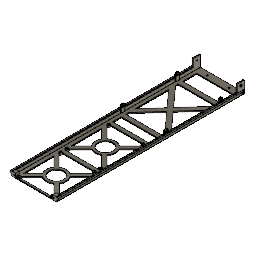
1-CBA_slide_tray_assembly_v11 (Autodesk Fusion 360 design; units mm, degrees)
Autodesk Fusion 360 part; units mm, degrees
sketch "Main Profile" plane through (0, 0, 0) normal (0, 1, 0) x (1, 0, 0)
  line L0 (0, 0) -> (62.1, 0)
  line L1 (62.1, 0) -> (62.1, -5.4)
  line L2 (62.1, -5.4) -> (66.55, -5.4)
  line L3 (66.55, -5.4) -> (66.55, -11.15)
  line L4 (66.55, -11.15) -> (62.1, -11.15)
  line L5 (62.1, -11.15) -> (62.1, -11.6)
  line L6 (62.1, -11.6) -> (58.7, -11.6)
  line L7 (58.7, -11.6) -> (58.7, -2.95)
  line L8 (58.7, -2.95) -> (0, -2.95)
  line L9 (0, -2.95) -> (0, 0) construction
  line L10 (0, 0) -> (-62.1, 0)
  line L11 (-62.1, 0) -> (-62.1, -5.4)
  line L12 (-62.1, -5.4) -> (-66.55, -5.4)
  line L13 (-66.55, -5.4) -> (-66.55, -11.15)
  line L14 (-66.55, -11.15) -> (-62.1, -11.15)
  line L15 (-62.1, -11.15) -> (-62.1, -11.6)
  line L16 (-62.1, -11.6) -> (-58.7, -11.6)
  line L17 (-58.7, -11.6) -> (-58.7, -2.95)
  line L18 (-58.7, -2.95) -> (0, -2.95)
  line L19 (60.6, -12.45) -> (50.6, -12.45)
  line L20 (50.6, -12.45) -> (50.6, -2.95)
  line L21 (60.6, -11.6) -> (60.6, -12.45)
  circle A0 centre (54.4, -6.11) radius 1.75
  circle A1 centre (54.4, -6.11) radius 2.5
  circle A2 centre (-54.4, -6.11) radius 1.75
  circle A3 centre (-54.4, -6.11) radius 2.5
  line L22 (-50.6, -12.45) -> (-50.6, -2.95)
  line L23 (-60.6, -12.45) -> (-50.6, -12.45)
  line L24 (-60.6, -11.6) -> (-60.6, -12.45)
  dimension "d1" = 2.95
  dimension "d2" = 5.75
  dimension "d3" = 5.4
  dimension "d4" = 4.45
  dimension "d5" = 62.1
  dimension "d6" = 11.6
  dimension "d7" = 3.4
  dimension "d10" = 10
  dimension "d11" = 9.5
  dimension "d12" = 50.6
  dimension "d13" = 3.5
  dimension "d14" = 5
  dimension "d15" = 3.16
  dimension "d16" = 54.4
  constraint coincident L0.start L9.end
  constraint horizontal L0
  constraint perpendicular L0 L1
  constraint perpendicular L1 L2
  constraint perpendicular L2 L3
  constraint perpendicular L3 L4
  constraint perpendicular L4 L5
  constraint perpendicular L5 L6
  constraint perpendicular L6 L7
  constraint perpendicular L7 L8
  constraint vertical L9
  constraint symmetric L0.start L9 L10.start
  constraint symmetric L0.end L9 L10.end
  constraint symmetric L1.end L9 L11.end
  constraint symmetric L2.end L9 L12.end
  constraint symmetric L3.end L9 L13.end
  constraint symmetric L4.end L9 L14.end
  constraint symmetric L5.end L9 L15.end
  constraint symmetric L6.end L9 L16.end
  constraint symmetric L7.end L9 L17.end
  constraint symmetric L8.end L9 L18.end
  constraint horizontal L19
  constraint vertical L20
  constraint vertical L21
  constraint coincident L6 L21.start
  constraint coincident L8 L20.end
  constraint concentric A0 A1
  constraint collinear L1 L5
  constraint symmetric L9 L19.start L23.start
  constraint symmetric L9 L19.end L22.start
  constraint symmetric L9 L20.end L22.end
  constraint symmetric L9 L21.start L24.start
  constraint symmetric L9 A0 A2
  constraint symmetric L9 A1 A3
  measures "d1" distance of L0 L8
  measures "d2" distance of L2 L4
  measures "d3" distance of L0 L2
  measures "d4" distance of L1 L3
  measures "d5" distance of L0.start L1
  measures "d6" distance of L0 L6
  measures "d7" distance of L1 L7
  measures "d10" distance of L19.start L19.end
  measures "d11" distance of L8 L19
  measures "d12" distance of L0.start L20
  measures "d13" diameter of A0
  measures "d14" diameter of A1
  measures "d15" distance of L8 A0.centre
  measures "d16" horizontal distance of L8.end A0.centre
extrude "Extrude1" add sketch "Main Profile" along normal blind 515.25 contours L0 L1 L2 L3 L4 L5 L6 L7 L8 L10 L11 L12 L13 L14 L15 L16 L17 L18
extrude "Extrude2" add sketch "Main Profile" along normal blind 10 contours L6 L7 L8 L19 L20 L21 | L16 L17 L18 L22 L23 L24
extrude "Extrude3" add sketch "Main Profile" along normal blind 5 contours A1 | A3
sketch "Solver says NO" plane through (0, 0, 0) normal (0, 0, 1) x (1, 0, 0)
  circle A0 centre (45.9, 4.2) radius 4
  circle A1 centre (45.9, 4.2) radius 2.5
  circle A2 centre (45.9, 4.2) radius 1.75
  circle A3 centre (0, 61) radius 20
  circle A4 centre (0, 61) radius 27.5
  circle A5 centre (-46.134, 4.2) radius 1.75
  circle A6 centre (-46.134, 4.2) radius 2.5
  circle A7 centre (-46.134, 4.2) radius 4
  circle A8 centre (45.9, 119.158) radius 1.75
  circle A9 centre (45.9, 119.158) radius 2.5
  circle A10 centre (45.9, 119.158) radius 4
  circle A11 centre (-46.134, 119.158) radius 1.75
  circle A12 centre (-46.134, 119.158) radius 2.5
  circle A13 centre (-46.134, 119.158) radius 4
  line L0 (-42.261, 5.2) -> (42.027, 5.2)
  line L1 (15.6223, 38.3683) -> (45.8401, 8.1996)
  line L2 (0, 61) -> (0, 50.5957) construction
  line L3 (-15.6446, 38.3837) -> (-45.8374, 8.189)
  line L4 (-23.2581, 46.3266) -> (-49, 20.5831)
  line L5 (-49, 20.5831) -> (-49, 102.9438)
  line L6 (-49, 102.9438) -> (-22.6501, 76.5956)
  line L7 (49, 102.9438) -> (22.6501, 76.5956)
  line L8 (49, 20.5831) -> (49, 102.9438)
  line L9 (23.2581, 46.3266) -> (49, 20.5831)
  line L10 (-14.7242, 84.226) -> (-45.6836, 115.1834)
  line L11 (-43.5366, 122.2) -> (43.3026, 122.2)
  line L12 (45.6651, 115.1649) -> (14.7242, 84.226)
  circle A14 centre (-46.134, 251.182) radius 1.75
  circle A15 centre (-46.134, 251.182) radius 2.5
  circle A16 centre (-46.134, 251.182) radius 4
  circle A17 centre (45.9, 251.182) radius 1.75
  circle A18 centre (45.9, 251.182) radius 2.5
  circle A19 centre (45.9, 251.182) radius 4
  circle A20 centre (45.9, 136.224) radius 1.75
  circle A21 centre (45.9, 136.224) radius 2.5
  circle A22 centre (45.9, 136.224) radius 4
  circle A23 centre (-46.134, 136.224) radius 1.75
  circle A24 centre (-46.134, 136.224) radius 2.5
  circle A25 centre (-46.134, 136.224) radius 4
  circle A26 centre (0, 195.782) radius 20
  circle A27 centre (0, 195.782) radius 27.5
  line L13 (-43.5157, 133.2) -> (43.2817, 133.2)
  line L14 (-44.8891, 140.0253) -> (-13.3101, 171.7177)
  line L15 (44.885, 140.0931) -> (13.3101, 171.7177)
  line L16 (21.6973, 178.8859) -> (49.0009, 151.5393)
  line L17 (49.0292, 234.0867) -> (24.0397, 209.1365)
  line L18 (49, 234.1286) -> (49, 151.5391)
  line L19 (-49.0292, 234.0867) -> (-24.0397, 209.1365)
  line L20 (-49, 234.1286) -> (-49, 151.5391)
  line L21 (-21.6973, 178.8859) -> (-49.0009, 151.5393)
  line L22 (-46.6162, 247.2112) -> (-16.8934, 217.4814)
  line L23 (16.8372, 217.525) -> (46.595, 247.2428)
  line L24 (-43.3759, 254.079) -> (43.1419, 254.079)
  line L25 (-49.2095, 288.349) -> (48.9656, 288.349)
  line L26 (48.9656, 288.349) -> (48.9656, 265.1555)
  line L27 (48.9656, 265.1555) -> (-49.2095, 265.1555)
  line L28 (-49.2095, 265.1555) -> (-49.2095, 288.349)
  line L29 (0.0587, 363.2451) -> (48.9913, 308.7576)
  line L30 (48.9913, 308.7576) -> (48.9913, 301.474)
  line L31 (48.9913, 301.474) -> (-49.1967, 301.474)
  line L32 (-49.1967, 301.474) -> (-49.1967, 308.5361)
  line L33 (-49.1967, 308.5361) -> (0.0587, 363.2451)
  line L34 (48.9892, 444.3369) -> (48.9892, 437.1705)
  line L35 (48.9892, 437.1705) -> (-0.0024, 382.821)
  line L36 (-0.0024, 382.821) -> (-49.2156, 437.4742)
  line L37 (-49.2156, 437.4742) -> (-49.2156, 444.3429)
  line L38 (-49.2156, 444.3429) -> (48.9892, 444.3369)
  line L39 (-8.8518, 372.9976) -> (-49.2156, 328.1276)
  line L40 (-49.2156, 328.1276) -> (-49.2102, 417.8091)
  line L41 (-49.2102, 417.8091) -> (-8.8518, 372.9976)
  line L42 (8.8407, 372.9976) -> (48.9641, 328.447)
  line L43 (48.9641, 328.447) -> (48.9694, 417.5445)
  line L44 (48.9694, 417.5445) -> (8.8407, 372.9976)
  line L45 (-49.2077, 495.2626) -> (48.9405, 495.2626)
  line L46 (48.9405, 495.2626) -> (48.9405, 457.4496)
  line L47 (48.9405, 457.4496) -> (-49.2077, 457.4496)
  line L48 (-49.2077, 457.4496) -> (-49.2077, 495.2626)
  circle A28 centre (-30.0176, 505.2429) radius 1.75
  circle A29 centre (-30.0176, 505.2429) radius 3.5
  circle A30 centre (29.9824, 505.2429) radius 1.75
  circle A31 centre (29.9824, 505.2429) radius 3.5
  dimension "d21" = 8
  dimension "d22" = 5
  dimension "d23" = 3.5
  dimension "d24" = 45.9
  dimension "d25" = 40
  dimension "d26" = 61
  dimension "d27" = 55
  dimension "d30" = -92.034
  dimension "d31" = 114.958
  dimension "d32" = 4.2
  dimension "d33" = 5.2
  dimension "d34" = 11
  dimension "d35" = 49
  dimension "d37" = 11
  dimension "d38" = 117
  dimension "d39" = 11
  dimension "d42" = 0
  dimension "d43" = 132.024
  dimension "d46" = 0
  dimension "d47" = 134.782
  dimension "d49" = 11
  dimension "d50" = 11
  dimension "d51" = 3.5
  dimension "d52" = 7
  dimension "d55" = 60
  dimension "d56" = 0
  constraint concentric A0 A1
  constraint concentric A0 A2
  constraint vertical origin A3.centre
  constraint concentric A3 A4
  constraint coincident A7 L0.start
  constraint coincident A0 L0.end
  constraint horizontal L0
  constraint coincident A4 L1.start
  constraint coincident A0 L1.end
  constraint coincident A3.centre A4.centre
  constraint vertical L2
  constraint coincident A4 L3.start
  constraint coincident A7 L3.end
  constraint coincident A4 L4.start
  constraint parallel L3 L4
  constraint vertical L5
  constraint coincident A4 L6.end
  constraint perpendicular L4 L6
  constraint symmetric L2 L4.start L9.start
  constraint symmetric L2 L4.end L8.start
  constraint symmetric L2 L5.end L7.start
  constraint symmetric L2 L6.end L7.end
  constraint coincident A4 L10.start
  constraint coincident A13 L10.end
  constraint parallel L6 L10
  constraint coincident A13 L11.start
  constraint coincident A10 L11.end
  constraint horizontal L11
  constraint coincident A10 L12.start
  constraint coincident A4 L12.end
  constraint parallel L7 L12
  constraint horizontal L13
  constraint coincident A25 L13.start
  constraint coincident A22 L13.end
  constraint coincident A25 L14.start
  constraint coincident A27 L14.end
  constraint coincident A22 L15.start
  constraint coincident A27 L15.end
  constraint coincident A27 L16.start
  constraint parallel L15 L16
  constraint coincident A27 L17.end
  constraint perpendicular L15 L17
  constraint vertical L18
  constraint collinear L8 L18
  constraint symmetric L2 L16.start L21.start
  constraint symmetric L2 L16.end L21.end
  constraint symmetric L2 L17.start L19.start
  constraint symmetric L2 L17.end L19.end
  constraint symmetric L2 L18.start L20.start
  constraint symmetric L2 L18.end L20.end
  constraint coincident A16 L22.start
  constraint coincident A27 L22.end
  constraint coincident A27 L23.start
  constraint coincident A19 L23.end
  constraint coincident A16 L24.start
  constraint coincident A19 L24.end
  constraint horizontal L25
  constraint vertical L26
  constraint horizontal L27
  constraint vertical L28
  constraint vertical L30
  constraint perpendicular L30 L31
  constraint perpendicular L31 L32
  constraint parallel L32 L34
  constraint parallel L34 L37
  constraint perpendicular L38 L40
  constraint parallel L41 L42
  constraint parallel L40 L43
  constraint horizontal L45
  constraint vertical L46
  constraint horizontal L47
  constraint vertical L48
  constraint concentric A28 A29
  measures "d21" diameter of A0
  measures "d22" diameter of A1
  measures "d23" diameter of A2
  measures "d24" horizontal distance of origin A0.centre
  measures "d25" diameter of A3
  measures "d26" distance of origin A3.centre
  measures "d27" diameter of A4
  measures "d32" vertical distance of origin A0.centre
  measures "d33" distance of origin L0
  measures "d34" distance of L3 L4
  measures "d35" distance of origin L5
  measures "d37" distance of L6 L10
  measures "d38" distance of L0 L11
  measures "d39" distance of L7 L12
  measures "d49" distance of L11 L13
  measures "d50" distance of L15 L16
  measures "d51" diameter of A28
  measures "d52" diameter of A29
extrude "Extrude4" cut sketch "Solver says NO" along normal blind 31.628 contours A0 A4 A7 L0 L1 L3 | A4 L7 L8 L9 | A4 L4 L5 L6 | A4 A10 A13 L10 L11 L12 | A2 | A3 | A5 | A8 | A11 | A14 | A16 A19 A27 L22 L23 L24 | A27 L19 L20 L21 | A27 L16 L17 L18 | A22 A25 A27 L13 L14 L15 | A17 | A20 | A23 | A26 | L25 L26 L27 L28 | L29 L30 L31 L32 L33 | L34 L35 L36 L37 L38 | L39 L40 L41 | L42 L43 L44 | L45 L46 L47 L48 | A28 | A30
extrude "Extrude5" add sketch "Solver says NO" along normal blind 5.5 contours A0 | A7 | A13 | A10 | A1 | A6 | A9 | A12 | A25 | A22 | A21 | A24
extrude "Extrude6" add sketch "Solver says NO" along normal blind 5 contours A15 | A16 | A19 | A18
extrude "Extrude7" cut sketch "Solver says NO" along normal blind 2.8 contours A1 | A6 | A9 | A12 | A21 | A24
extrude "Extrude8" cut sketch "Solver says NO" along normal blind 2.2 contours A15 | A18
extrude "Extrude9" cut sketch "Solver says NO" along normal blind 1 contours A29 | A31
sketch "Knobs" plane through (0, 0, 2.95) normal (0, 0, 1) x (-1, 0, 0)
  arc A0 (43.5366, -122.2) -> (45.6836, -115.1834) centre (46.134, -119.158) ccw
  line L0 (43.5366, -122.2) -> (-43.3026, -122.2)
  arc A1 (-45.6651, -115.1649) -> (-43.3026, -122.2) centre (-45.9, -119.158) ccw
  line L1 (-45.6651, -115.1649) -> (-14.7242, -84.226)
  arc A2 (-14.7242, -84.226) -> (14.7242, -84.226) centre (0, -61) ccw
  line L2 (14.7242, -84.226) -> (45.6836, -115.1834)
  line L3 (49, -102.9438) -> (22.6501, -76.5956)
  arc A3 (22.6501, -76.5956) -> (23.2581, -46.3266) centre (0, -61) ccw
  line L4 (23.2581, -46.3266) -> (49, -20.5831)
  line L5 (49, -20.5831) -> (49, -102.9438)
  arc A4 (44.8891, -140.0253) -> (43.5157, -133.2) centre (46.134, -136.224) ccw
  line L6 (44.8891, -140.0253) -> (13.3101, -171.7177)
  arc A5 (13.3101, -171.7177) -> (-13.3101, -171.7177) centre (0, -195.782) ccw
  line L7 (-13.3101, -171.7177) -> (-44.885, -140.0931)
  arc A6 (-43.2817, -133.2) -> (-44.885, -140.0931) centre (-45.9, -136.224) ccw
  line L8 (-43.2817, -133.2) -> (43.5157, -133.2)
  line L9 (49.1967, -308.5361) -> (-0.0587, -363.2451)
  line L10 (-0.0587, -363.2451) -> (-48.9913, -308.7576)
  line L11 (-48.9913, -308.7576) -> (-48.9913, -301.474)
  line L12 (-48.9913, -301.474) -> (49.1967, -301.474)
  line L13 (49.1967, -301.474) -> (49.1967, -308.5361)
  line L14 (49.2077, -457.4496) -> (49.2077, -495.2626)
  line L15 (49.2077, -495.2626) -> (-48.9405, -495.2626)
  line L16 (-48.9405, -495.2626) -> (-48.9405, -457.4496)
  line L17 (-48.9405, -457.4496) -> (49.2077, -457.4496)
  line L18 (49.2102, -417.8091) -> (8.8518, -372.9976)
  line L19 (8.8518, -372.9976) -> (49.2156, -328.1276)
  line L20 (49.2156, -328.1276) -> (49.2102, -417.8091)
  arc A7 (-21.6973, -178.8859) -> (-24.0397, -209.1365) centre (0, -195.782) ccw
  line L21 (-24.0397, -209.1365) -> (-49, -234.0576)
  line L22 (-49, -234.0576) -> (-49, -151.5402)
  line L23 (-49, -151.5402) -> (-21.6973, -178.8859)
  arc A8 (-23.2581, -46.3266) -> (-22.6501, -76.5956) centre (0, -61) ccw
  line L24 (-22.6501, -76.5956) -> (-49, -102.9438)
  line L25 (-49, -102.9438) -> (-49, -20.5831)
  line L26 (-49, -20.5831) -> (-23.2581, -46.3266)
  circle A9 centre (-29.9824, -505.2429) radius 1.75
  circle A10 centre (0, -61) radius 20
  line L27 (49, -234.0576) -> (24.0397, -209.1365)
  arc A11 (24.0397, -209.1365) -> (21.6973, -178.8859) centre (0, -195.782) ccw
  line L28 (21.6973, -178.8859) -> (49, -151.5402)
  line L29 (49, -151.5402) -> (49, -234.0576)
  circle A12 centre (0, -195.782) radius 20
  line L30 (-48.9694, -417.5445) -> (-48.9641, -328.447)
  line L31 (-48.9641, -328.447) -> (-8.8407, -372.9976)
  line L32 (-8.8407, -372.9976) -> (-48.9694, -417.5445)
  line L33 (49.2156, -444.3429) -> (-48.9892, -444.3369)
  line L34 (-48.9892, -444.3369) -> (-48.9892, -437.1705)
  line L35 (-48.9892, -437.1705) -> (0.0024, -382.821)
  line L36 (0.0024, -382.821) -> (49.2156, -437.4742)
  line L37 (49.2156, -437.4742) -> (49.2156, -444.3429)
  line L38 (49.2095, -265.1555) -> (49.2095, -288.349)
  line L39 (49.2095, -288.349) -> (-48.9656, -288.349)
  line L40 (-48.9656, -288.349) -> (-48.9656, -265.1555)
  line L41 (-48.9656, -265.1555) -> (49.2095, -265.1555)
  arc A13 (-42.027, -5.2) -> (-45.8401, -8.1996) centre (-45.9, -4.2) ccw
  line L42 (-42.027, -5.2) -> (42.261, -5.2)
  arc A14 (45.8374, -8.189) -> (42.261, -5.2) centre (46.134, -4.2) ccw
  line L43 (45.8374, -8.189) -> (15.6446, -38.3837)
  arc A15 (15.6446, -38.3837) -> (-15.6223, -38.3683) centre (0, -61) ccw
  line L44 (-15.6223, -38.3683) -> (-45.8401, -8.1996)
  circle A16 centre (30.0176, -505.2429) radius 1.75
  line L45 (50.6, -10) -> (50.6, 0)
  line L46 (50.6, 0) -> (-50.6, 0)
  line L47 (-50.6, 0) -> (-50.6, -10)
  line L48 (-50.6, -10) -> (-58.7, -10)
  line L49 (-58.7, -10) -> (-58.7, -515.25)
  line L50 (-58.7, -515.25) -> (58.7, -515.25)
  line L51 (58.7, -515.25) -> (58.7, -10)
  line L52 (58.7, -10) -> (50.6, -10)
  arc A17 (43.3759, -254.079) -> (46.6162, -247.2112) centre (46.134, -251.182) ccw
  line L53 (43.3759, -254.079) -> (-43.1419, -254.079)
  arc A18 (-46.595, -247.2428) -> (-43.1419, -254.079) centre (-45.9, -251.182) ccw
  line L54 (-46.595, -247.2428) -> (-16.8372, -217.525)
  arc A19 (-16.8372, -217.525) -> (16.8934, -217.4814) centre (0, -195.782) ccw
  line L55 (16.8934, -217.4814) -> (46.6162, -247.2112)
  line L56 (61.6, -307.5) -> (57.5, -307.5)
  line L57 (57.5, -307.5) -> (57.5, -295.5)
  line L58 (57.5, -295.5) -> (61.6, -295.5)
  line L59 (61.6, -295.5) -> (61.6, -307.5)
  line L60 (61.6, -445.5) -> (61.6, -457.5)
  line L61 (57.5, -445.5) -> (61.6, -445.5)
  line L62 (57.5, -457.5) -> (57.5, -445.5)
  line L63 (61.6, -457.5) -> (57.5, -457.5)
  line L64 (62.1, 0) -> (62.1, -515.25)
  line L65 (58.7, -495.25) -> (62.1, -495.25)
  line L66 (62.1, -515.25) -> (58.7, -515.25)
  line L67 (58.7, -10) -> (58.7, -515.25)
  dimension "d69" = 4.1
  dimension "d70" = 12
  dimension "d71" = 295.5
  dimension "d72" = 57.5
  dimension "d75" = 0
  dimension "d76" = -150
  dimension "d77" = 20
  constraint horizontal L56
  constraint vertical L57
  constraint horizontal L58
  constraint vertical L59
  constraint coincident L51 L65.start
  constraint coincident L64 L65.end
  constraint perpendicular L51 L65
  measures "d69" distance of L57 L59
  measures "d70" distance of L56 L58
  measures "d71" distance of origin L58
  measures "d72" distance of origin L57
  measures "d77" distance of L65 L66
extrude "Extrude10" add sketch "Knobs" along normal blind 30 contours L51 L64 L65 L66 L67
extrude "Extrude11" add sketch "Knobs" along normal blind 20 contours L51 L56 L58 L59 L67 | L51 L56 L57 L58 L67 | L51 L60 L61 L63 L67 | L51 L61 L62 L63 L67
sketch "Side Holes" plane through (-62.1, 0, 0) normal (-1, 0, 0) x (0, -1, 0)
  line L0 (-515.25, 11.15) -> (0, 11.15)
  line L1 (0, 11.15) -> (0, 11.6)
  line L2 (0, 11.6) -> (-495.25, 11.6)
  line L3 (-495.25, 11.6) -> (-495.25, 32.95)
  line L4 (-495.25, 32.95) -> (-515.25, 32.95)
  line L5 (-515.25, 32.95) -> (-515.25, 11.15)
  circle A0 centre (-505.25, 23.95) radius 3.5
  circle A1 centre (-505.25, 23.95) radius 1.75
  circle A2 centre (-451.5, 16.95) radius 2.5
  circle A3 centre (-451.5, 16.95) radius 4
  circle A4 centre (-301.5, 16.95) radius 2.5
  circle A5 centre (-301.5, 16.95) radius 4
  dimension "d82" = 7
  dimension "d83" = 3.5
  dimension "d84" = 10
  dimension "d85" = 9
  dimension "d86" = 5
  dimension "d87" = 8
  dimension "d88" = 16
  dimension "d89" = 63.75
  dimension "d92" = 150
  dimension "d93" = 0
  constraint concentric A0 A1
  constraint concentric A2 A3
  measures "d82" diameter of A0
  measures "d83" diameter of A1
  measures "d84" distance of L5 A0.centre
  measures "d85" distance of L4 A0.centre
  measures "d86" diameter of A2
  measures "d87" diameter of A3
  measures "d88" distance of L4 A2.centre
  measures "d89" distance of L5 A2.centre
extrude "Extrude12" cut sketch "Side Holes" against normal blind 1.4 contours A0
extrude "Extrude13" cut 1 faces at (-62.1, 504.551, 23.4174) along direction (1, 0, 0) blind 9.184
extrude "Extrude14" cut sketch "Side Holes" against normal blind 2.47 contours A3 | A5
extrude "Extrude15" cut sketch "Side Holes" against normal blind 17.71 contours A2 | A4
mirror "Mirror1" about plane through (0, 0, 0) normal (1, 0, 0) of "Extrude10", "Extrude11", "Extrude12", "Extrude13", "Extrude14", "Extrude15"
fillet "Fillet1" radius 5 8 edges at (59.55, 457.5, 22.95) (59.55, 445.5, 22.95) (-59.55, 445.5, 22.95) (-59.55, 457.5, 22.95) (-59.55, 295.5, 22.95) (-59.55, 307.5, 22.95) (59.55, 295.5, 22.95) (59.55, 307.5, 22.95)
fillet "Fillet2" radius 1 40 edges at (61.6, 295.5, 14.775) (61.6, 296.9645, 21.4855) (61.6, 301.5, 22.95) (61.6, 306.0355, 21.4855) (61.6, 307.5, 14.775) (57.5, 307.5, 10.45) (57.5, 306.0355, 21.4855) (57.5, 301.5, 22.95) (57.5, 296.9645, 21.4855) (57.5, 295.5, 10.45) (61.6, 445.5, 14.775) (61.6, 446.9645, 21.4855) (61.6, 451.5, 22.95) (61.6, 456.0355, 21.4855) (61.6, 457.5, 14.775) (57.5, 445.5, 10.45) (57.5, 446.9645, 21.4855) (57.5, 451.5, 22.95) (57.5, 456.0355, 21.4855) (57.5, 457.5, 10.45) (-57.5, 445.5, 10.45) (-57.5, 446.9645, 21.4855) (-57.5, 451.5, 22.95) (-57.5, 456.0355, 21.4855) (-57.5, 457.5, 10.45) (-61.6, 457.5, 14.775) (-61.6, 456.0355, 21.4855) (-61.6, 451.5, 22.95) (-61.6, 446.9645, 21.4855) (-61.6, 445.5, 14.775) (-61.6, 307.5, 14.775) (-61.6, 306.0355, 21.4855) (-61.6, 301.5, 22.95) (-61.6, 296.9645, 21.4855) (-61.6, 295.5, 14.775) (-57.5, 295.5, 10.45) (-57.5, 296.9645, 21.4855) (-57.5, 301.5, 22.95) (-57.5, 306.0355, 21.4855) (-57.5, 307.5, 10.45)
chamfer "Chamfer1" distance 4.45 distance2 12 2 edges at (66.55, 515.25, 8.275) (-66.55, 515.25, 8.275) measured on face at (59.8333, 515.25, 15.6833) measured on face at (59.8333, 515.25, 15.6833)
named bodies: "1-CBA_slide_tray_assembly_v11"
